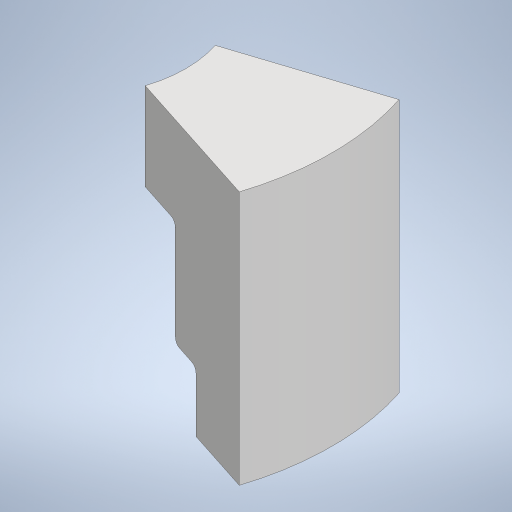
# Autodesk Inventor part: креп_подш
Saved by Autodesk Inventor 2023 (Build 270158000, 158)
## iProperties
Created: 2025-02-05
Part Number: креп_подш
Material: Типовые
Document SubType Name: Modeling
Designer: baranovaem
Density: 1 g/cm^3
Appearance: По умолчанию
Author: baranovaem
Autodesk Inventor part; units mm, degrees
ref_plane "YZ Plane" through (0, 0, 0) normal (1, 0, 0) x (0, 1, 0)
ref_plane "XZ Plane" through (0, 0, 0) normal (0, 1, 0) x (-1, 0, 0)
ref_plane "XY Plane" through (0, 0, 0) normal (0, 0, 1) x (1, 0, 0)
sketch "Эскиз3" plane through (0, 0, 0) normal (0, 0, 1) x (1, 0, 0)
  line L0 (28.4814, 0) -> (32, 0)
  line L1 (26.4814, 18.1962) -> (19.4814, 18.1962)
  line L2 (19.4814, 18.1962) -> (19.4814, 33.1962)
  line L3 (27.4814, 17.1962) -> (27.4814, 1)
  line L4 (33, -1) -> (33, -10.35)
  line L5 (33, -10.35) -> (44.4955, -10.35)
  line L6 (109.4355, -10.35) -> (-108.0344, -10.35) projected
  arc A0 (33, -1) -> (32, 0) centre (32, -1) ccw
  arc A1 (27.4814, 1) -> (28.4814, 0) centre (28.4814, 1) ccw
  arc A2 (27.4814, 17.1962) -> (26.4814, 18.1962) centre (26.4814, 17.1962) ccw
  line L7 (19.4814, 33.1962) -> (44.4955, 33.1962)
  line L8 (44.4955, 33.1962) -> (44.4955, -10.35)
  point P0 (27.4814, 18.1962)
  point P1 (27.4814, 0)
  dimension "d25" = 8
  dimension "d42" = 15
  dimension "d44" = 1
  dimension "d45" = 1
  dimension "d54" = 3.5186
  dimension "d55" = 25.0142
  constraints: 16 end point, 6 point on circle, 6 tangent, 4 point on line, 3 centre point, 3 horizontal, 3 perpendicular, 2 vertical, 1 equal radius
  measures "d25" distance of L1.end point (27.481, 18.196)
  measures "d42" distance of L1.end L2.end
  measures "d44" radius of A0
  measures "d45" radius of A2
  measures "d54" distance of L0.start L0.end
  measures "d55" distance between parallel lines of L2 L8
sketch "Эскиз4" plane through (0, 0, 0) normal (0, 1, 0) x (-1, 0, 0)
  arc A0 (-24.7386, 8) -> (-24.7386, -8) centre (0, 0) ccw
  dimension "d31" = 26
  constraints: 2 point on circle, 1 centre point
  measures "d31" radius of A0
sweep "Сдвиг1" add profiles "Эскиз3" path "Эскиз4"
sketch "Эскиз8" plane through (0, -10.35, 0) normal (0, -1, 0) x (1, 0, 0)
  arc A0 (31.399, -10.1538) -> (31.399, 10.1538) centre (0, 0) ccw projected
  arc A1 (35.205, -11.3846) -> (35.205, 11.3846) centre (0, 0) ccw construction
  line L0 (42.3369, -13.6909) -> (31.399, -10.1538) projected
  circle A2 centre (36.723, -4.5186) radius 1.575
  circle A3 centre (36.723, 4.5186) radius 1.575
  line L1 (31.399, 10.1538) -> (42.3369, 13.6909) projected
  point P0 (0, 0)
  dimension "d46" = 4
  dimension "d47" = 3.15
  dimension "d48" = 3.15
  dimension "d49" = 7
  dimension "d50" = 7
  constraints: 4 point on circle, 3 centre point
  measures "d46" radial gap between concentric circles of A0 A1
  measures "d47" diameter of A2
  measures "d48" diameter of A3
  measures "d49" distance from line of L0 A2.centre
  measures "d50" distance from line of A3.centre L1
extrude "Выдавливание4" cut sketch "Эскиз8" against normal blind 10
